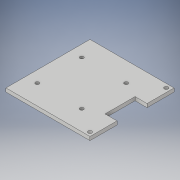
# Autodesk Inventor part: 000.107 - Правая стенка среднего сегмента
Saved by Autodesk Inventor 2019 (Build 230136000, 136)
## iProperties
Created: 2020-06-06
Part Number: 000.107 - Правая стенка среднего сегмента
Material: Типовые
Document SubType Name: Modeling
Designer: Петров Иван
Density: 1 g/cm^3
Appearance: По умолчанию
Author: Петров Иван
Autodesk Inventor part; units mm, degrees
ref_plane "YZ Plane" through (0, 0, 0) normal (1, 0, 0) x (0, 1, 0)
ref_plane "XZ Plane" through (0, 0, 0) normal (0, 1, 0) x (-1, 0, 0)
ref_plane "XY Plane" through (0, 0, 0) normal (0, 0, 1) x (1, 0, 0)
sketch "Эскиз1" plane through (0, 0, 0) normal (0, 1, 0) x (-1, 0, 0)
  line L0 (-35, 35) -> (35, 35)
  line L1 (35, 35) -> (35, -35)
  line L2 (35, -35) -> (-35, -35)
  line L3 (-35, -35) -> (-35, 35)
  line L4 (-35, 35) -> (35, -35) construction
  line L5 (35, 35) -> (-35, -35) construction
  line L6 (-35, 35) -> (-31.7678, 31.7678)
  circle A0 centre (-31.7678, 31.7678) radius 1.6
  line L7 (-35, -35) -> (-31.7678, -31.7678)
  circle A1 centre (-31.7678, -31.7678) radius 1.6
  point P0 (0, 0)
  dimension "d0" = 70
  dimension "d1" = 70
  dimension "d2" = 4.571
  dimension "d3" = 3.2
  dimension "d4" = 4.571
  dimension "d5" = 3.2
  constraints: 16 end point, 2 centre point, 2 coincident, 2 midpoint, 2 parallel, 2 point on line, 1 horizontal, 1 perpendicular
  measures "d0" distance of L1.end L2.end
  measures "d1" distance of L0.end L1.end
  measures "d2" distance of L0.start L6.end
  measures "d3" diameter of A0
  measures "d4" distance of L2.end L7.end
  measures "d5" diameter of A1
extrude "Выдавливание1" add sketch "Эскиз1" along normal blind 3
sketch "Эскиз2" plane through (35, 0, 35) normal (1, 0, 0) x (0, 0, -1)
  line L0 (35, 0) -> (35, 3)
  line L1 (0, 3) -> (70, 3) projected
  line L2 (22.5, 0) -> (47.5, 0)
  line L3 (47.5, 0) -> (47.5, 3)
  line L4 (47.5, 3) -> (22.5, 3)
  line L5 (22.5, 3) -> (22.5, 0)
  line L6 (22.5, 0) -> (47.5, 3) construction
  line L7 (47.5, 0) -> (22.5, 3) construction
  point P0 (35, 1.5)
  dimension "d8" = 25
  constraints: 14 end point, 4 midpoint, 2 parallel, 1 horizontal, 1 perpendicular, 1 point on line
  measures "d8" distance of L4.end L3.end
extrude "Выдавливание2" cut sketch "Эскиз2" against normal blind 10
sketch "Эскиз3" plane through (0, 3, 0) normal (0, 1, 0) x (1, 0, 0)
  line L0 (-28.375, -21.875) -> (-28.375, 21.875)
  line L1 (14.625, -21.875) -> (-28.375, -21.875)
  line L2 (14.625, 21.875) -> (14.625, -21.875)
  line L3 (-28.375, 21.875) -> (14.625, 21.875)
  circle A0 centre (11.625, -18.5) radius 1.5
  circle A1 centre (-25.375, -18.5) radius 1.5
  circle A2 centre (-25.375, 18.5) radius 1.5
  circle A3 centre (11.625, 18.5) radius 1.5
  point P0 (0, 0)
  point P1 (-6.875, 0)
  constraints: 8 end point, 4 centre point
extrude "Выдавливание3" cut sketch "Эскиз3" against normal blind 10 contours A0 | A1 | A2 | A3
equation "\"d4\" = d2"
equation "\"d5\" = d3"
